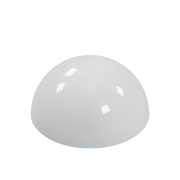
# Autodesk Inventor part: 11_Range
Saved by Autodesk Inventor 2022 (Build 260153000, 153)
## iProperties
Created: 2022-06-10
Part Number: 11_Range
Material: Generic
Document SubType Name: Modeling
Designer: pzach
Density: 1 g/cm^3
Appearance: Sky Blue Medium
Author: pzach
Autodesk Inventor part; units mm, degrees
ref_plane "YZ Plane" through (0, 0, 0) normal (1, 0, 0) x (0, 1, 0)
ref_plane "XZ Plane" through (0, 0, 0) normal (0, 1, 0) x (-1, 0, 0)
ref_plane "XY Plane" through (0, 0, 0) normal (0, 0, 1) x (1, 0, 0)
sketch "Sketch2" plane through (0, 0, 0) normal (1, 0, 0) x (0, 1, 0)
  arc A0 (0, -3000) -> (0, 3000) centre (0, 0) ccw
  line L0 (0, -3000) -> (0, 3000)
  dimension "d2" = 6000
  dimension "d3" = 6000
  constraints: 2 end point, 2 point on circle, 1 centre point, 1 coincident, 1 vertical
  measures "d2" diameter of A0
  measures "d3" distance of L0.start L0.end
extrude "Extrusion1" add sketch "Sketch2" along normal mid plane 6000
fillet "Fillet1" radius 3000 2 edges at (3000, 3000, 0) (-3000, 3000, 0)
body "Solid1"
